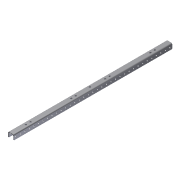
# Autodesk Inventor part: C Channel 1764
Saved by Autodesk Inventor 2011 (Build 150239000, 239)
## iProperties
Created: 2009-01-11
Part Number: C Channel 1764
Document SubType Name: Modeling
Designer: jrobinson
Density: 1 g/cm^3
Author: jrobinson
Autodesk Inventor part; units mm, degrees
ref_plane "YZ Plane" through (0, 0, 0) normal (1, 0, 0) x (0, 1, 0)
ref_plane "XZ Plane" through (0, 0, 0) normal (0, 1, 0) x (-1, 0, 0)
sketch "Sketch1" plane through (0, 0, 0) normal (0, 0, 1) x (1, 0, 0)
  line L0 (-25.9259, -4.2593) -> (-25.9259, 24.3157)
  line L1 (-25.9259, 24.3157) -> (5.8241, 24.3157)
  line L2 (5.8241, 24.3157) -> (5.8241, -4.2593)
  line L3 (5.8241, -4.2593) -> (2.6491, -4.2593)
  line L4 (2.6491, -4.2593) -> (2.6491, 21.1407)
  line L5 (2.6491, 21.1407) -> (-22.7509, 21.1407)
  line L6 (-22.7509, 21.1407) -> (-22.7509, -4.2593)
  line L7 (-22.7509, -4.2593) -> (-25.9259, -4.2593)
  dimension "d0" = 25.4
  dimension "d1" = 31.75
  dimension "d2" = 3.175
  dimension "d3" = 3.175
  dimension "d4" = 28.575
  dimension "d5" = 0
  constraints: 16 end point, 6 parallel, 1 perpendicular, 1 vertical
  measures "d0" distance between parallel lines of L4 L6
  measures "d1" distance between parallel lines of L0 L2
  measures "d2" distance between parallel lines of L2 L4
  measures "d3" distance between parallel lines of L1 L5
  measures "d4" distance between parallel lines of L1 L3
  measures "d5" distance between parallel lines of L7 L3
extrude "Extrusion1" add sketch "Sketch1" along normal blind 889
fillet "Fillet1" radius 6.35 4 edges at (-22.7509, 21.1407, 444.5) (-25.9259, 24.3157, 444.5) (5.8241, 24.3157, 444.5) (2.6491, 21.1407, 444.5)
fillet "Fillet2" radius 3.175 4 edges at (4.2366, -4.2593, 889) (-24.3384, -4.2593, 889) (-24.3384, -4.2593, 0) (4.2366, -4.2593, 0)
sketch "Sketch2" plane through (-25.9259, 17.9657, 0) normal (-1, 0, 0) x (0, 0, 1)
  line L0 (3.175, -22.225) -> (885.825, -22.225) projected
  line L1 (0, -19.05) -> (0, 0) projected
  circle A0 centre (12.7, -9.525) radius 3.175
  dimension "d10" = 6.35
  dimension "d11" = 12.7
  dimension "d12" = 12.7
  constraints: 1 centre point
  measures "d10" diameter of A0
  measures "d11" distance from line of L0 A0.centre
  measures "d12" distance from line of L1 A0.centre
extrude "Extrusion2" cut sketch "Sketch2" against normal through all
pattern_linear "Rectangular Pattern1" count 35 spacing 25.4 along (0, 0, 1) of "Extrusion2"
sketch "Sketch3" plane through (-19.5759, 24.3157, 0) normal (0, 1, 0) x (1, 0, 0)
  line L0 (0, -889) -> (19.05, -889) projected
  circle A0 centre (11.1125, -806.45) radius 4.7625
  line L1 (25.4, -3.175) -> (25.4, -885.825) projected
  dimension "d18" = 9.525
  dimension "d20" = 82.55
  dimension "d30" = 14.2875
  constraints: 1 centre point
  measures "d18" diameter of A0
  measures "d20" distance from line of L0 A0.centre
  measures "d30" distance from line of L1 A0.centre
extrude "Extrusion3" cut sketch "Sketch3" against normal through all
pattern_linear "Rectangular Pattern2" count 2 spacing 25.4 along (0, 0, -1) of "Extrusion3"
pattern_linear "Rectangular Pattern3" count 2 spacing 254 along (0, 0, -1) of "Extrusion3", "Rectangular Pattern2"
ref_plane "Work Plane2" through (67.878, 24.3157, 444.5) normal (0, 0, -1) x (-1, 0, 0)
mirror "Mirror1" about plane through (67.878, 24.3157, 444.5) normal (0, 0, -1) of "Extrusion3", "Rectangular Pattern2", "Rectangular Pattern3"
sketch "Sketch5" plane through (-19.5759, 24.3157, 0) normal (0, 1, 0) x (1, 0, 0)
  line L0 (0, 0) -> (19.05, 0) projected
  circle A0 centre (7.9375, -444.5) radius 4.7625
  line L1 (-6.35, -3.175) -> (-6.35, -885.825) projected
  dimension "d31" = 9.525
  dimension "d32" = 14.2875
  dimension "d33" = 444.5
  constraints: 1 centre point
  measures "d31" diameter of A0
  measures "d32" distance from line of L1 A0.centre
  measures "d33" distance from line of L0 A0.centre
extrude "Extrusion4" cut sketch "Sketch5" against normal through all
sketch "Sketch8" plane through (5.8241, 17.9657, 889) normal (1, 0, 0) x (0, 0, -1)
  circle A0 centre (12.7, -9.525) radius 3.175 projected
  circle A1 centre (38.1, -9.525) radius 3.175 projected
  circle A2 centre (63.5, -9.525) radius 3.175 projected
  circle A3 centre (88.9, -9.525) radius 3.175 projected
  circle A4 centre (114.3, -9.525) radius 3.175 projected
  circle A5 centre (139.7, -9.525) radius 3.175 projected
  circle A6 centre (165.1, -9.525) radius 3.175 projected
  circle A7 centre (190.5, -9.525) radius 3.175 projected
  circle A8 centre (215.9, -9.525) radius 3.175 projected
  circle A9 centre (241.3, -9.525) radius 3.175 projected
  circle A10 centre (266.7, -9.525) radius 3.175 projected
  circle A11 centre (292.1, -9.525) radius 3.175 projected
  circle A12 centre (317.5, -9.525) radius 3.175 projected
  circle A13 centre (342.9, -9.525) radius 3.175 projected
  circle A14 centre (368.3, -9.525) radius 3.175 projected
  circle A15 centre (393.7, -9.525) radius 3.175 projected
  circle A16 centre (419.1, -9.525) radius 3.175 projected
  circle A17 centre (444.5, -9.525) radius 3.175 projected
  circle A18 centre (469.9, -9.525) radius 3.175 projected
  circle A19 centre (495.3, -9.525) radius 3.175 projected
  circle A20 centre (520.7, -9.525) radius 3.175 projected
  circle A21 centre (546.1, -9.525) radius 3.175 projected
  circle A22 centre (571.5, -9.525) radius 3.175 projected
  circle A23 centre (596.9, -9.525) radius 3.175 projected
  circle A24 centre (622.3, -9.525) radius 3.175 projected
  circle A25 centre (647.7, -9.525) radius 3.175 projected
  circle A26 centre (673.1, -9.525) radius 3.175 projected
  circle A27 centre (698.5, -9.525) radius 3.175 projected
  circle A28 centre (723.9, -9.525) radius 3.175 projected
  circle A29 centre (749.3, -9.525) radius 3.175 projected
  circle A30 centre (774.7, -9.525) radius 3.175 projected
  circle A31 centre (800.1, -9.525) radius 3.175 projected
  circle A32 centre (825.5, -9.525) radius 3.175 projected
  circle A33 centre (850.9, -9.525) radius 3.175 projected
  circle A34 centre (876.3, -9.525) radius 3.175 projected
  arc A35 (885.825, -22.225) -> (889, -19.05) centre (885.825, -19.05) ccw projected
  line L0 (889, 0) -> (889, -19.05) projected
  line L1 (0, 0) -> (889, 0) projected
  line L2 (0, 0) -> (0, -19.05) projected
  arc A36 (0, -19.05) -> (3.175, -22.225) centre (3.175, -19.05) ccw projected
  line L3 (885.825, -22.225) -> (3.175, -22.225) projected
  point P0 (889, -17.9657)
body "Solid1"
